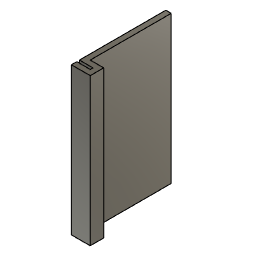
side_holder (Autodesk Fusion 360 design; units mm, degrees)
Autodesk Fusion 360 part; units mm, degrees
sketch "Sketch1" plane through (0, 0, 0) normal (0, 0, 1) x (1, 0, 0)
  line L0 (-3.5, 17.5) -> (3.5, 17.5)
  line L1 (3.5, 17.5) -> (3.5, -17.5)
  line L2 (3.5, -17.5) -> (-3.5, -17.5)
  line L3 (-3.5, -17.5) -> (-3.5, 17.5)
  line L4 (-3.5, 17.5) -> (3.5, -17.5) construction
  line L5 (3.5, 17.5) -> (-3.5, -17.5) construction
  dimension "d13" = 7
  dimension "d14" = 35
  constraint horizontal L0
  constraint perpendicular L0 L1
  constraint parallel L0 L2
  constraint parallel L1 L3
  constraint coincident L4 origin
  constraint coincident L5 origin
  measures "d13" distance of L1.end L2.end
  measures "d14" distance of L0.end L1.end
extrude "Extrude1" add sketch "Sketch1" along normal blind 54.6
sketch "Sketch2" plane through (0, 0, 54.6) normal (0, 0, 1) x (-1, 0, 0)
  line L0 (3.5, 17.5) -> (-3.5, 17.5)
  line L1 (-3.5, 17.5) -> (-3.5, -17.5)
  line L2 (-3.5, -17.5) -> (3.5, -17.5)
  line L3 (3.5, -17.5) -> (3.5, 17.5)
  line L4 (-3.5, -17.5) -> (1.5, -17.5)
  line L5 (1.5, -17.5) -> (1.5, 12.5)
  line L6 (1.5, 12.5) -> (-3.5, 12.5)
  line L7 (-3.5, 12.5) -> (-3.5, -17.5)
  dimension "d17" = 5
  dimension "d18" = 30
  constraint horizontal L4
  constraint vertical L5
  constraint horizontal L6
  constraint vertical L7
  constraint coincident L1.end L2.start
  measures "d17" distance of L1.end L4.end
  measures "d18" distance of L1.end L6.end
extrude "Extrude2" cut sketch "Sketch2" against normal blind 54.6 contours L1 L2 L4 L5 L6 L7
sketch "Sketch3" plane through (0, 0, 54.6) normal (0, 0, 1) x (-1, 0, 0)
  line L0 (1.5, 12.5) -> (1.5, -17.5)
  line L1 (1.5, -17.5) -> (3.5, -17.5)
  line L2 (3.5, -17.5) -> (3.5, 17.5)
  line L3 (3.5, 17.5) -> (-3.5, 17.5)
  line L4 (-3.5, 17.5) -> (-3.5, 12.5)
  line L5 (-3.5, 12.5) -> (1.5, 12.5)
  line L6 (-1.5, 14.5) -> (3.5, 14.5)
  line L7 (3.5, 14.5) -> (3.5, 15.5)
  line L8 (3.5, 15.5) -> (-1.5, 15.5)
  line L9 (-1.5, 15.5) -> (-1.5, 14.5)
  dimension "d21" = 5
  dimension "d22" = 1
  constraint horizontal L6
  constraint vertical L7
  constraint horizontal L8
  constraint vertical L9
  measures "d21" distance of L6.start L6.end
  measures "d22" distance of L6.start L8.end
extrude "Extrude3" cut sketch "Sketch3" against normal blind 54.6 contours L2 L6 L7 L8 L9
